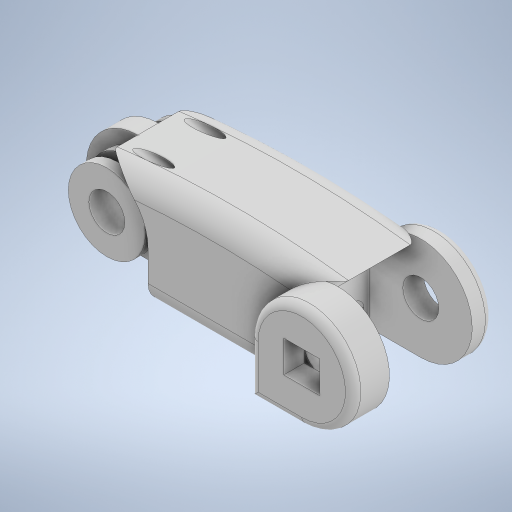
# Autodesk Inventor part: BottomPart
Saved by Autodesk Inventor 2024 (Build 280153000, 153)
## iProperties
Created: 2024-03-20
Part Number: BottomPart
Material: Generic
Document SubType Name: Modeling
Designer: Wojtek
Density: 1 g/cm^3
Appearance: Default
Author: Wojtek
Autodesk Inventor part; units mm, degrees
ref_plane "YZ Plane" through (0, 0, 0) normal (1, 0, 0) x (0, 1, 0)
sketch "Sketch1" plane through (0, 0, 0) normal (0, 0, 1) x (1, 0, 0)
  line L0 (0, 20) -> (45, 20)
  line L1 (0, 0) -> (0, 20)
  arc A0 (45, 20) -> (35, 10) centre (45, 10) ccw
  line L2 (35, 10) -> (35, 0)
  circle A1 centre (45, 10) radius 10
  circle A2 centre (45, 10) radius 3.5
  line L3 (0, 0) -> (45, 0)
  circle A3 centre (0, 10) radius 10
  circle A4 centre (0, 10) radius 3.5
  arc A5 (45, 20) -> (0, 20) centre (22.5, -158.588213) ccw
  line L4 (10, 10) -> (10, 0)
  circle A6 centre (0, 10) radius 7.5
  circle A7 centre (0, 10) radius 3.5
  circle A8 centre (45, 10) radius 3.5
  dimension "d0" = 45
  dimension "d1" = 20
  dimension "d2" = 10
  dimension "d4" = 45
  dimension "d5" = 7
  dimension "d6" = 20
  dimension "d7" = 7
  dimension "d9" = 180
  dimension "d14" = 15
  dimension "d47" = 7
  dimension "d48" = 7
  constraints: 10 end point, 9 centre point, 8 point on circle, 6 coincident, 3 tangent, 2 perpendicular, 1 horizontal, 1 midpoint, 1 point on line, 1 vertical
  measures "d0" distance of L0.start L0.end
  measures "d1" diameter of A0
  measures "d2" distance of L2.start L2.end
  measures "d4" horizontal distance of A0.centre L1.start
  measures "d5" diameter of A2
  measures "d6" diameter of A3
  measures "d7" diameter of A4
  measures "d9" radius of A5
  measures "d14" diameter of A6
  measures "d47" diameter of A7
  measures "d48" diameter of A8
extrude "Extrusion1" add sketch "Sketch1" along normal mid plane 20 contours A5 L0 | L0 A0 L2 L3 L4 A3
extrude "Extrusion2" add sketch "Sketch1" along normal mid plane 4 contours A3 L1 A6 | L1 A6 A3 | A1 A0 | A6 L1 A4 | L1 A4 A6 | L4 L3 A3 | A1 L3 L2
extrude "Extrusion3" add sketch "Sketch1" along normal mid plane 8 contours A6 L1 A4 | L1 A4 A6
sketch "Sketch2" plane through (0, 10, 4) normal (0, 0, 1) x (1, 0, 0)
  circle A0 centre (0, 0) radius 6
  circle A1 centre (0, 0) radius 7.5 projected
  circle A2 centre (0, 0) radius 3.5
  point P0 (0, -10)
  dimension "d17" = 12
  dimension "d18" = 1.5
  dimension "d19" = 7
  constraints: 2 centre point, 1 coincident
  measures "d17" diameter of A0
  measures "d18" radial gap between concentric circles of A1 A0
  measures "d19" diameter of A2
extrude "Extrusion4" add sketch "Sketch2" along normal blind 2 contours A0
sketch "Sketch3" plane through (0, 10, 6) normal (0, 0, 1) x (1, 0, 0)
  circle A0 centre (0, 0) radius 7.5
  circle A1 centre (0, 0) radius 6
  circle A2 centre (0, 0) radius 3.5 projected
  point P0 (0, -10)
  dimension "d22" = 15
  dimension "d23" = 12
  dimension "d24" = 2.5
  constraints: 2 centre point, 1 coincident
  measures "d22" diameter of A0
  measures "d23" diameter of A1
  measures "d24" radial gap between concentric circles of A2 A1
extrude "Extrusion5" add sketch "Sketch3" along normal blind 2 contours A0 | A1
sketch "Sketch4" plane through (0, 10, -4) normal (0, 0, -1) x (-1, 0, 0)
  circle A0 centre (0, 0) radius 6
  circle A1 centre (0, 0) radius 3.5 projected
  point P0 (0, -10)
  dimension "d27" = 12
  dimension "d28" = 2.5
  constraints: 1 centre point
  measures "d27" diameter of A0
  measures "d28" radial gap between concentric circles of A1 A0
extrude "Extrusion6" add sketch "Sketch4" along normal blind 2
sketch "Sketch5" plane through (0, 10, -6) normal (0, 0, -1) x (-1, 0, 0)
  circle A0 centre (0, 0) radius 3.5 projected
  circle A1 centre (0, 0) radius 7.5
  point P0 (0, -10)
  dimension "d31" = 15
  constraints: 1 centre point, 1 coincident
  measures "d31" diameter of A1
extrude "Extrusion7" add sketch "Sketch5" along normal blind 2
extrude "Extrusion8" add sketch "Sketch1" along normal mid plane 22 contours A1 A0 | A1 L3 L2
extrude "Extrusion9" cut sketch "Sketch1" along normal mid plane 16.1 contours A1 A0 | A1 L3 L2 | A2
sketch "Sketch6" plane through (0, 0, 0) normal (0, 0, 1) x (1, 0, 0)
  line L0 (0, 20) -> (25, 20)
  line L1 (0, 0) -> (0, 20)
  circle A0 centre (0, 10) radius 10
  circle A1 centre (25, 10) radius 10
  line L2 (0, 0) -> (25, 0)
  line L3 (10, 10) -> (10, 0)
  line L4 (15, 10) -> (15, 0)
  circle A2 centre (0, 10) radius 3.5
  circle A3 centre (25, 10) radius 3.5
  dimension "d39" = 25
  dimension "d40" = 20
  dimension "d41" = 20
  dimension "d42" = 25
  dimension "d43" = 7
  dimension "d44" = 7
  constraints: 10 end point, 5 point on circle, 4 centre point, 3 tangent, 2 coincident, 2 perpendicular, 2 point on line, 1 horizontal, 1 midpoint, 1 vertical
  measures "d39" distance of L0.start L0.end
  measures "d40" distance from line of L1.start L0
  measures "d41" diameter of A1
  measures "d42" distance of L1.start L2.end
  measures "d43" diameter of A2
  measures "d44" diameter of A3
fillet "Fillet1" radius 4 4 edges at (22.5, 21.4118, 10) (22.5, 21.4118, -10) (22.5, 0, 10) (22.5, 0, -10)
fillet "Fillet2" radius 1 6 edges at (35, 5, 11) (40, 0, 11) (52.0711, 17.0711, 11) (40, 0, -11) (35, 5, -11) (52.0711, 17.0711, -11)
extrude "Extrusion10" cut sketch "Sketch1" along normal mid plane 20 contours A4 L1 | L1 A4 | A2
extrude "Extrusion11" cut sketch "Sketch1" along normal mid plane 25 contours A2
extrude "Extrusion12" add sketch "Sketch1" along normal mid plane 24.2 contours A1 A0 | A1 L3 L2
extrude "Extrusion13" cut sketch "Sketch1" along normal mid plane 16.1 contours A1 A0 | A1 L3 L2
fillet "Fillet3" radius 1.5 6 edges at (35, 5, 12.1) (40, 0, 12.1) (52.0711, 17.0711, 12.1) (52.0711, 17.0711, -12.1) (40, 0, -12.1) (35, 5, -12.1)
sketch "Sketch8" plane through (35, 0.565251, -8.05) normal (1, 0, 0) x (0, 0, -1)
  line L0 (-4.05, 3.434749) -> (-2.05, 3.434749)
  line L1 (-12.05, 3.434749) -> (-14.05, 3.434749)
  circle A0 centre (-13.05, 3.434749) radius 1
  circle A1 centre (-3.05, 3.434749) radius 1
  line L2 (-12.05, 15.434749) -> (-14.05, 15.434749)
  line L3 (-4.05, 15.434749) -> (-2.05, 15.434749)
  circle A2 centre (-13.05, 15.434749) radius 1
  circle A3 centre (-3.05, 15.434749) radius 1
  point P0 (-8.05, -0.565251)
  dimension "d58" = 2
  dimension "d59" = 2
  constraints: 4 coincident, 4 midpoint, 3 horizontal alignment, 1 centre point, 6 other
  measures "d59" diameter of A1
ref_plane "Work Plane1" through (35, 4, -5) normal (0, 0, 1) x (1, 0, 0)
ref_plane "Work Plane2" through (35, 4, 5) normal (0, 0, 1) x (1, 0, 0)
sketch "Sketch9" plane through (35, 4, 5) normal (0, 0, 1) x (1, 0, 0)
  line L0 (0, 0) -> (-25, -4)
  line L1 (0, 0) -> (0, 6) construction
  line L2 (0, 6) -> (-20.87433, 6) construction
  line L3 (0, 12) -> (-25, 16)
  line L4 (-25, 16) -> (-40.64391, 18.503026)
  line L5 (0, 12) -> (17.116469, 9.261365)
  point P0 (-35, -4)
  dimension "d68" = 25
  dimension "d69" = 4
  dimension "d70" = 6
  dimension "d71" = 25
  dimension "d72" = 15.64391
  dimension "d73" = 9.09028
  dimension "d78" = 17.11647
  dimension "d79" = 9.09028
  constraints: 12 end point, 2 symmetric about line, 1 horizontal, 1 vertical
  measures "d68" horizontal distance of L0.start L0.end
  measures "d69" vertical distance of L0.start L0.end
  measures "d70" distance of L0.start L1.end
  measures "d71" horizontal distance of L3.start L3.end
  measures "d72" horizontal distance of L3.end L4.end
  measures "d73" angle of L2 L4
  measures "d78" horizontal distance of L3.start L5.end
  measures "d79" angle of L2 L5
sketch "Sketch10" plane through (35, 4, -5) normal (0, 0, 1) x (1, 0, 0)
  line L0 (0, 0) -> (-25, -4)
  line L1 (0, 0) -> (0, 12) construction
  line L2 (0, 6) -> (-16.940116, 6) construction
  line L3 (0, 12) -> (-25, 16)
  line L4 (-25, 16) -> (-43.341178, 18.934588)
  line L5 (0, 12) -> (17.085345, 9.266345)
  point P0 (-35, -4)
  dimension "d64" = 12
  dimension "d74" = 18.34118
  dimension "d75" = 9.09028
  dimension "d80" = 17.08534
  dimension "d81" = 9.09028
  constraints: 12 end point, 1 horizontal, 1 midpoint, 1 symmetric about line, 1 vertical
  measures "d64" distance of L0.start L1.end
  measures "d74" horizontal distance of L3.end L4.end
  measures "d75" angle of L2 L4
  measures "d80" horizontal distance of L1.end L5.end
  measures "d81" angle of L2 L5
sweep "Sweep1" cut profiles "Sketch8" path "Sketch9" path curves L0 contours A1 L0 | L0 A1 | A0 L1 | L1 A0
fillet "Fillet4" radius 1 2 edges at (10, 1, -5) (10, 1, 5)
fillet "Fillet5" radius 1 2 edges at (35, 4, 6) (35, 4, -4)
sweep "Sweep2" cut profiles "Sketch8" path "Sketch10" path curves L3 L4 contours A2 L2 | L2 A2 | A3 L3 | L3 A3
sweep "Sweep3" cut profiles "Sketch8" path "Sketch9" path curves L5 L3 L4 contours A2 L2 | L2 A2 | A3 L3 | L3 A3
fillet "Fillet6" radius 2 2 edges at (36.8161, 15.7467, 5.9993) (36.8161, 15.7467, -4.0007)
sketch "Sketch12" plane through (0, 0, 12.1) normal (0, 0, 1) x (1, 0, 0)
  circle A0 centre (45, 10) radius 3.5 projected
  circle A1 centre (45, 10) radius 3.5
  circle A2 centre (45, 10) radius 10
  line L0 (36.5, 1.5) -> (35, 0) projected
  line L1 (35, 10) -> (35, 0)
  line L2 (35, 0) -> (45, 0)
  point P0 (0, 0)
  dimension "d85" = 7
  constraints: 4 end point, 2 centre point, 2 coincident, 2 point on circle, 2 tangent, 1 vertical
  measures "d85" diameter of A1
extrude "Extrusion14" add sketch "Sketch12" along normal blind 3 and the other way blind 2.5
fillet "Fillet7" radius 1.5 3 edges at (35, 5, 15.1) (40, 0, 15.1) (52.0711, 17.0711, 15.1)
sketch "Sketch13" plane through (0, 0, 15.1) normal (0, 0, 1) x (1, 0, 0)
  circle A0 centre (45, 10) radius 3.5 projected
  circle A1 centre (45, 10) radius 5
  line L0 (41.5, 6.9) -> (48.5, 6.9)
  line L1 (48.5, 6.9) -> (48.5, 13.1)
  line L2 (48.5, 13.1) -> (41.5, 13.1)
  line L3 (41.5, 13.1) -> (41.5, 6.9)
  line L4 (41.5, 6.9) -> (48.5, 13.1) construction
  line L5 (48.5, 6.9) -> (41.5, 13.1) construction
  point P0 (0, 0)
  dimension "d91" = 10
  dimension "d92" = 7
  dimension "d93" = 6.2
  constraints: 12 end point, 2 midpoint, 2 parallel, 1 centre point, 1 coincident, 1 horizontal, 1 perpendicular
  measures "d91" diameter of A1
  measures "d92" distance of L2.end L1.end
  measures "d93" distance of L1.end L0.end
extrude "Extrusion15" add sketch "Sketch13" against normal blind 4 contours A0 L0 L2 | L1 L0 A0 | A0 L2 L1 | L2 A0 | A0 L0 | A0 L3 L2 | L0 L3 A0 | A1
extrude "Extrusion16" cut sketch "Sketch13" against normal blind 4 contours A0 L0 L2 | L1 L0 A0 | A0 L2 L1 | A0 L3 L2 | L0 L3 A0
body "Solid1"
